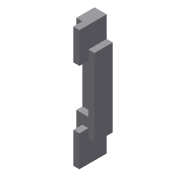
# Autodesk Inventor part: Tunnel_Holder
Saved by Autodesk Inventor 2016 (Build 200138000, 138)
## iProperties
Created: 2016-11-30
Part Number: Tunnel_Holder
Material: Generic
Document SubType Name: Modeling
Designer: reinert
Density: 1 g/cm^3
Appearance: Default
Author: reinert
Autodesk Inventor part; units mm, degrees
ref_plane "YZ Plane" through (0, 0, 0) normal (1, 0, 0) x (0, 1, 0)
ref_plane "XZ Plane" through (0, 0, 0) normal (0, 1, 0) x (-1, 0, 0)
ref_plane "XY Plane" through (0, 0, 0) normal (0, 0, 1) x (1, 0, 0)
sketch "Sketch1" plane through (0, 0, 0) normal (0, 1, 0) x (-1, 0, 0)
  line L0 (0, 0) -> (10, 0)
  line L1 (10, 0) -> (10, -128)
  line L2 (10, -128) -> (0, -128)
  line L3 (0, -128) -> (0, 0)
  line L4 (10, -128) -> (10, -163)
  line L5 (10, -163) -> (30, -163)
  line L6 (10, 0) -> (10, 35)
  line L7 (10, 35) -> (30, 35)
  line L8 (30, 35) -> (30, -163)
  dimension "d16" = 35
  dimension "d17" = 20
  dimension "d18" = 35
  dimension "d19" = 20
  dimension "d28" = 128
  dimension "d35" = 10
  constraints: 18 end point, 3 perpendicular, 2 parallel, 1 horizontal, 1 point on line, 1 vertical
  measures "d16" distance of L1.end L4.end
  measures "d17" distance of L4.end L5.end
  measures "d18" distance of L0.end L6.end
  measures "d19" distance of L6.end L7.end
  measures "d28" distance of L2.end L0.start
  measures "d35" distance of L0.start L0.end
extrude "Extrusion1" add sketch "Sketch1" along normal blind 30
sketch "Sketch2" plane through (0, 0, 0) normal (0, -1, 0) x (1, 0, 0)
  line L0 (-30, -163) -> (-30, 35) projected
  line L1 (-30, -104) -> (-10, -104)
  line L2 (-10, -104) -> (-10, -24)
  line L3 (-10, -24) -> (-30, -24)
  line L4 (-30, -24) -> (-30, -104)
  line L5 (-10, 0) -> (0, 0) projected
  dimension "d22" = 20
  dimension "d23" = 80
  dimension "d25" = 24
  constraints: 8 end point, 2 parallel, 1 horizontal, 1 perpendicular, 1 point on line
  measures "d22" distance of L3.end L2.end
  measures "d23" distance of L2.end L1.end
  measures "d25" distance from line of L5 L2.end
extrude "Extrusion6" cut sketch "Sketch2" against normal blind 10
sketch "Sketch6" plane through (0, 0, 0) normal (0, -1, 0) x (1, 0, 0)
  line L0 (-30, -24) -> (-10, -24) projected
  line L1 (-10, 0) -> (0, 0) projected
  line L2 (-30, -24) -> (0, -24)
  line L3 (0, -24) -> (0, 0)
  line L4 (0, 0) -> (-30, 0)
  line L5 (-30, 0) -> (-30, -24)
  line L6 (-10, -104) -> (-30, -104) projected
  line L7 (0, 0) -> (0, -128) projected
  line L8 (-30, -104) -> (0, -104)
  line L9 (0, -104) -> (0, -128)
  line L10 (0, -128) -> (-30, -128)
  line L11 (-30, -128) -> (-30, -104)
  constraints: 16 end point, 4 parallel, 2 horizontal, 2 perpendicular
extrude "Extrusion7" add sketch "Sketch6" along normal blind 30
body "Solid1"
